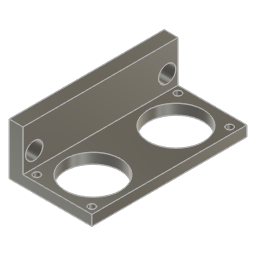
Ultrasonic Sensor Baseplate v4 (Autodesk Fusion 360 design; units mm, degrees)
Autodesk Fusion 360 part; units mm, degrees
sketch "Sketch1" plane through (0, 0, 0) normal (0, 0, 1) x (1, 0, 0)
  line L0 (0, 0) -> (20, 0)
  line L1 (20, 0) -> (20, 45)
  line L2 (20, 45) -> (0, 45)
  line L3 (0, 45) -> (0, 0)
  circle A0 centre (9.8866, 34.5367) radius 8
  circle A1 centre (10.1679, 10.139) radius 8
  circle A2 centre (2, 43) radius 1
  circle A3 centre (18, 42) radius 1
  circle A4 centre (18, 2) radius 1
  circle A5 centre (2, 2) radius 1
  point P0 (2, 43)
  dimension "d1" = 20
  dimension "d2" = 45
  dimension "d3" = 16
  dimension "d4" = 16
  constraint horizontal L0
  constraint vertical L1
  constraint horizontal L2
  constraint vertical L3
  constraint coincident L0.start L3.end
  measures "d1" distance of L0.start L0.end
  measures "d2" distance of L0.start L2.end
  measures "d3" diameter of A0
  measures "d4" diameter of A1
extrude "Extrude1" add sketch "Sketch1" along normal blind 2
sketch "Sketch2" plane through (0, 0, 0) normal (1, 0, 0) x (0, 1, 0)
  line L0 (0, 0) -> (45, 0)
  line L1 (45, 0) -> (45, 15)
  line L2 (45, 15) -> (0, 15)
  line L3 (0, 15) -> (0, 0)
  circle A0 centre (3.2668, 7.4482) radius 2.5
  circle A1 centre (41.8901, 7.426) radius 2.5
  dimension "d7" = 5
  dimension "d8" = 5
  constraint horizontal L0
  constraint vertical L1
  constraint horizontal L2
  constraint vertical L3
  constraint coincident L0.start L3.end
  measures "d7" diameter of A0
  measures "d8" diameter of A1
extrude "Extrude2" add sketch "Sketch2" against normal blind 1
sketch "Sketch3" plane through (0, 0, 2) normal (0, 0, 1) x (-1, 0, 0)
  circle A0 centre (-2, -2) radius 1
  circle A1 centre (-18, -2) radius 1
  circle A2 centre (-10.1679, -10.139) radius 8
  circle A3 centre (-18, -42) radius 1
  circle A4 centre (-9.8866, -34.5367) radius 8
  circle A5 centre (-2, -43) radius 1
  line L0 (0, -45) -> (0, 0)
  line L1 (0, 0) -> (-20, 0)
  line L2 (-20, 0) -> (-20, -45)
  line L3 (-20, -45) -> (0, -45)
extrude "Extrude3" add 1 faces at (-1, 16.6085, 13.1343) along direction (-1, 0, 0) blind 3
extrude "Extrude4" add sketch "Sketch3" along normal blind 1
